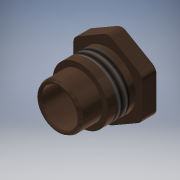
# Autodesk Inventor part: Packing Nut
Saved by Autodesk Inventor 2018 (Build 220112000, 112)
## iProperties
Shininess: 64.0
Length Units: 11269
Angle Units: 11279
Time Units: 11290
Mass Units: 11283
Length Display Precision: 3
Angle Display Precision: 2
Compacted: True
Part Number: Packing Nut
Document SubType Name: Modeling
Created: 2003-04-15
Designer: James M. Leake
Material: Bronze, Soft Tin
Density: 8.874 g/cm^3
Appearance: Bronze - Satin
Density: 0.0
Volumn: 0.0
Area: 0.0
PropertySet Name: Model Information
Control State: 0
Master: False
Checked Out: False
Author: James M. Leake
Autodesk Inventor part; units mm, degrees
ref_plane "YZ Plane" through (0, 0, 0) normal (1, 0, 0) x (0, 1, 0)
ref_plane "XZ Plane" through (0, 0, 0) normal (0, 1, 0) x (-1, 0, 0)
ref_plane "XY Plane" through (0, 0, 0) normal (0, 0, 1) x (1, 0, 0)
sketch "Sketch1" plane through (0, 0, 0) normal (0, 0, 1) x (1, 0, 0)
  line L0 (-1, 0) -> (13, 0) projected
  line L1 (0, -2.3) -> (0, 29.9) projected
  line L2 (6.5, 0) -> (6.5, 18)
  line L3 (6.5, 18) -> (8.5, 18)
  line L4 (8.5, 18) -> (8.5, 21)
  line L5 (8.5, 21) -> (6.5, 21)
  line L6 (6.5, 21) -> (6.5, 23)
  line L7 (6.5, 23) -> (10, 23)
  line L8 (10, 23) -> (10, 8)
  line L9 (10, 8) -> (8, 8)
  line L10 (8, 8) -> (8, 0)
  line L11 (8, 0) -> (6.5, 0)
  point P0 (0, 0)
  dimension "d0" = 13
  dimension "d1" = 16
  dimension "d2" = 20
  dimension "d3" = 8
  dimension "d4" = 23
  dimension "d5" = 2
  dimension "d6" = 3
  dimension "d7" = 2
  constraints: 20 end point, 6 parallel, 3 perpendicular, 2 collinear, 2 point on line
  measures "d0" diameter of L2 L1
  measures "d1" diameter of L10 L1
  measures "d2" diameter of L8 L1
  measures "d3" distance of L9.end L10.end
  measures "d4" distance between parallel lines of L7 L0
  measures "d5" distance of L5.end L6.end
  measures "d6" distance of L3.end L4.end
  measures "d7" distance of L2.end L3.end
revolve "Revolution1" add sketch "Sketch1" angle 360 about axis through (0, -10, 0) along (0, 1, 0)
sketch "Sketch2" plane through (0, 23, 0) normal (0, 1, 0) x (1, 0, 0)
  circle A0 centre (0, 0) radius 10 projected
  circle A1 centre (0, 0) radius 6.5 projected
  line L0 (-12, 0) -> (16, 0) projected
  line L1 (0, 12) -> (0, -16) projected
  line L2 (0, -14.4338) -> (-12.5, -7.2169)
  line L3 (-12.5, -7.2169) -> (-12.5, 7.2169)
  line L4 (-12.5, 7.2169) -> (0, 14.4338)
  line L5 (0, 14.4338) -> (12.5, 7.2169)
  line L6 (12.5, 7.2169) -> (12.5, -7.2169)
  line L7 (12.5, -7.2169) -> (0, -14.4338)
  dimension "d9" = 25
  constraints: 12 end point, 1 coincident, 1 point on line, 11 other
  measures "d9" distance between parallel lines of L6 L3
extrude "Extrusion1" add sketch "Sketch2" against normal blind 5 contours L0 L6 L7 L1 A0 | A0 L1 L2 L3 L4 L5 L6 L0
fillet "Fillet1" radius 3 6 edges at (0, 20.5, 14.4338) (-12.5, 20.5, 7.2169) (-12.5, 20.5, -7.2169) (0, 20.5, -14.4338) (12.5, 20.5, -7.2169) (12.5, 20.5, 7.2169)
chamfer "Chamfer1" distance 0.5 angle 45 1 edges at (-6.5, 0, 0)
chamfer "Chamfer2" distance 0.5 distance2 1 1 edges at (-8, 0, 0) measured on face at (7.5214, 0, 1.1966)
thread "Thread1" size "M20x2.5" class "6g" standard "ANSI Metric M Profile" length 5 offset 3
body "Solid1"
